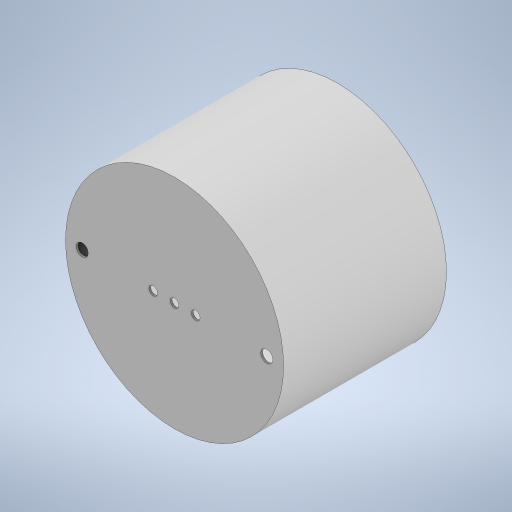
# Autodesk Inventor part: outer vessel
Saved by Autodesk Inventor 2023 (Build 270158000, 158)
## iProperties
Created: 2023-01-25
Part Number: outer vessel
Material: Generic
Document SubType Name: Modeling
Designer: remidm
Density: 1 g/cm^3
Appearance: Default
Mass: 16.5116 g
Surface Area: 331.292 cm^2
Volume: 16.5116 cm^3
Author: remidm
Autodesk Inventor part; units mm, degrees
ref_plane "YZ Plane" through (0, 0, 0) normal (1, 0, 0) x (0, 1, 0)
ref_plane "XZ Plane" through (0, 0, 0) normal (0, 1, 0) x (-1, 0, 0)
ref_plane "XY Plane" through (0, 0, 0) normal (0, 0, 1) x (1, 0, 0)
sketch "Sketch1" plane through (0, 0, 0) normal (0, 0, 1) x (1, 0, 0)
  circle A0 centre (0, 0) radius 62.8175
  dimension "OuterVesselInnerdiameter" = 125.635
  constraints: 1 centre point, 1 coincident
  measures "OuterVesselInnerdiameter" diameter of A0
extrude "Extrusion1" add sketch "Sketch1" along normal blind 93.8496
shell "Shell2" thickness 1 removed faces 0
sketch "Sketch2" plane through (0, 0, 93.8496) normal (0, 0, 1) x (1, 0, 0)
  line L0 (0, 0) -> (-12.25, 0)
  line L1 (0, 0) -> (12.25, 0)
  point P0 (53.194, 0)
  point P1 (-53.194, 0)
  dimension "d21" = 53.194
  dimension "d22" = 53.194
  dimension "d30" = 24.5
  constraints: 4 end point, 2 horizontal, 1 collinear
  measures "d21" distance of L0.start point (-53.194, 0)
  measures "d22" distance of point (53.194, 0) L0.start
  measures "d30" distance of L1.end L0.end
hole "Hole1" at (-12.25, 0, 93.8496) at (0, 0, 93.8496) at (12.25, 0, 93.8496) direction (0, 0, -1) diameter 5 depth 1 tip angle 118
hole "Hole2" at (53.194, 0, 93.8496) at (-53.194, 0, 93.8496) direction (0, 0, -1) diameter 7 depth 1 tip angle 118
equation "\"OuterVesselInnerdiameter\" = 2.5 * CrucibleThickness + 2.5 * CrucibleInnerDiameter"
equation "\"height\" = 1.2 * SupportHeight + 1.2 * crucible_height"
equation "\"d21\" = OuterVesselBottomHolesSpacing"
equation "\"d22\" = OuterVesselBottomHolesSpacing"
equation "\"d30\" = DistanceBetweenHolesSweep"
equation "\"d14\" = PenetrationOuterDiameter"
equation "\"d23\" = PenetrationUpstreamInnerDiameter + 2 * PenetrationUpstreamThickness"
equation "\"OuterVesselTopHolesSpacing\" = DistanceBetweenHolesSweep"
equation "\"CrucibleThickness\" = 0.254"
equation "\"crucible_height\" = 68.208"
equation "\"CrucibleDistanceBetweenTopHoles\" = 7.62"
equation "\"OuterVesselBottomHolesSpacing\" = CrucibleThickness + 0.5 * CrucibleInnerDiameter + PenetrationUpstreamDistanceFromWallToCentre"
equation "\"CrucibleInnerDiameter\" = 50"
equation "\"SupportHeight\" = 10"
equation "\"DistanceBetweenHolesSweep\" = 24.499987"
equation "\"PenetrationOuterDiameter\" = 5"
equation "\"PenetrationUpstreamInnerDiameter\" = 5"
equation "\"PenetrationUpstreamThickness\" = 1"
equation "\"PenetrationUpstreamDistanceFromWallToCentre\" = 27.94"
body "Solid1"
